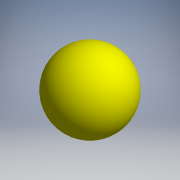
# Autodesk Inventor part: 15-40-19.1-12-ybrg2-124-6.747-28.5
Saved by Autodesk Inventor 2017.3 (Build 213256000, 256)
## iProperties
Part Number: 15-40-19.1-12-ybrg2-124-6.747-28.5
Material: Generic
Catalog Web Link: www.cadenas.de
Description: Ball for Y units-Y-bearings
Vendor: SKF
Document SubType Name: Modeling
Designer: partserver
Manufacturer: SKF
Mass: 0.160817 g
Surface Area: 1.43012 cm^2
Volume: 0.160817 cm^3
Density: 1 g/cm^3
Appearance: PSOLRGB-255-255-0
Category: PARTsolutions
Company: SKF
Title: 15-40-19.1-12-ybrg2-124-6.747-28.5
Author: Cadenas PARTsolutions
Comments: Y-bearings
PSOL_IDENT_0: {$CADENAS_DATA\23d-libs\skf\bearings_units_and_housings\bearing_units\ball_bearing_units\y-unit_acce
PSOL_IDENT_1: ssories\ball.prj},220 {VTYP=3D},{NB=15-40-19.1-12-ybrg2-124-6.747-28.5},{LINA=15-40-19.1-12-ybrg2-12
PSOL_IDENT_2: 4-6.747-28.5},{NN=Ball for Y units},{DATE=20.08.2020 13:45:09},{GEOMDATE=29.07.2020 16:06:32},{VERSI
PSOL_IDENT_3: ON=},{LINEID=2150},{WBVAR=},{WBNUMERIC=}  {NB=15-40-19.1-12-ybrg2-124-6.747-28.5},{LINA=15-40-19.1-1
PSOL_IDENT_4: 2-ybrg2-124-6.747-28.5},{KT=DUMMY},{DD=15.0000},{D=40},{B=19.100},{C=12.000},{PITCH=28.500},{DW=6.74
PSOL_IDENT_5: 7},{FO=IEC_BBY_005},{DESIGN=ybrg2},{X=0},{PN=124}
NB: 15-40-19.1-12-ybrg2-124-6.747-28.5
NN: Ball for Y units
NT: Y-bearings
NBSYN: $DD.-$D.-$B.-$C.-$DESIGN.-$PN.-$DW.-$PITCH.
LINA: 15-40-19.1-12-ybrg2-124-6.747-28.5
CATALOG: SKF
DD: 15
D: 40
B: 19.1
C: 12
PITCH: 28.5
DW: 6.747
FO: IEC_BBY_005
DESIGN: ybrg2
SUPPLIER: SKF
ARTICLENO: 15-40-19.1-12-ybrg2-124-6.747-28.5
BOMINFO: 15-40-19.1-12-ybrg2-124-6.747-28.5
CREATOR: CADENAS GmbH
Autodesk Inventor part; units mm, degrees
ref_plane "YZ Plane" through (0, 0, 0) normal (1, 0, 0) x (0, 1, 0)
ref_plane "XZ Plane" through (0, 0, 0) normal (0, 1, 0) x (-1, 0, 0)
ref_plane "XY Plane" through (0, 0, 0) normal (0, 0, 1) x (1, 0, 0)
sketch "Sketch_4" plane through (0, 0, 0) normal (0, 0, 1) x (1, 0, 0)
  line L0 (3.3735, 14.25) -> (-3.3735, 14.25)
  arc A0 (3.3735, 14.25) -> (-3.3735, 14.25) centre (0, 14.25) ccw
  line L1 (3.3735, 14.25) -> (-3.3735, 14.25)
  constraints: 4 end point, 2 point on circle, 1 centre point
revolve "Revolution1" add sketch "Sketch_4" angle 360 about axis through (3.3735, 14.25, 0) along (1, 0, 0)
ref_plane "ball_XY" through (0, 14.25, 0) normal (1, 0, 0) x (0, 0, -1)
ref_plane "ball_YZ" through (0, 14.25, 0) normal (0, 0, -1) x (0, 1, 0)
ref_plane "ball_ZX" through (0, 14.25, 0) normal (0, 1, 0) x (1, 0, 0)
body "Solid1"
